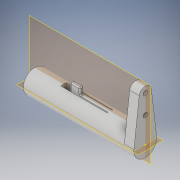
# Autodesk Inventor part: SR-T-07
Saved by Autodesk Inventor 2019.4 (Build 234330000, 330)
## iProperties
Created: 2019-06-15
Part Number: SR-T-07
Material: 一般
Document SubType Name: Modeling
Designer: Koki Shinjo
Mass: 0.853878 g
Surface Area: 9.79658 cm^2
Volume: 0.853878 cm^3
Density: 1 g/cm^3
Appearance: 既定
Author: Koki Shinjo
Autodesk Inventor part; units mm, degrees
ref_plane "YZ Plane" through (0, 0, 0) normal (1, 0, 0) x (0, 1, 0)
ref_plane "XY Plane" through (0, 0, 0) normal (0, 0, 1) x (1, 0, 0)
sketch "スケッチ1" plane through (0, 0, 0) normal (0, 0, 1) x (1, 0, 0)
  line L0 (0, 0) -> (0, 3)
  line L1 (0, 3) -> (-29, 3)
  line L2 (-29, 3) -> (-29, 0)
  line L3 (-29, 0) -> (0, 0)
  dimension "d0" = 29
  dimension "d1" = 3
  constraints: 8 end point, 3 perpendicular, 1 vertical
  measures "d0" distance of L0.end L1.end
  measures "d1" distance of L0.start L0.end
revolve "回転1" add sketch "スケッチ1" angle 360 about axis through (-29, 0, 0) along (1, 0, 0)
sketch "スケッチ2" plane through (0, 0, 0) normal (1, 0, 0) x (0, 0, -1)
  circle A0 centre (0, 6.7) radius 0.6
  circle A1 centre (0, 11.7) radius 0.6
  circle A2 centre (0, 11.7) radius 1.6
  line L0 (-1.5885, 11.8915) -> (-2.9784, 0.359)
  circle A3 centre (0, 0) radius 3 projected
  line L1 (2.9784, 0.359) -> (1.5885, 11.8915)
  dimension "d3" = 1.2
  dimension "d4" = 5
  dimension "d5" = 6.7
  dimension "d6" = 3.2
  constraints: 4 end point, 4 point on circle, 4 tangent, 3 centre point, 2 vertical alignment, 1 coincident, 1 equal radius
  measures "d3" diameter of A1
  measures "d4" distance of A1.centre A0.centre
  measures "d5" distance of point (0, 0) A0.centre
  measures "d6" diameter of A2
extrude "押し出し1" add sketch "スケッチ2" against normal blind 2.5 contours A2 | A2 L1 A3 L0
ref_plane "作業平面1" through (0, 0, 0) normal (0, 1, 0) x (-1, 0, 0)
sketch "スケッチ3" plane through (0, 0, 0) normal (0, 1, 0) x (-1, 0, 0)
  line L0 (0, 1.5885) -> (0, 2.9784) construction
  line L1 (0, 1.5885) -> (2.5, 1.5885) construction
  line L2 (2.5, 2.9784) -> (2.5, 1.5885) construction
  line L3 (2.5, 2.9784) -> (0, 2.9784) construction
  line L4 (0, 0.6) -> (2.5, 0.6) construction
  line L5 (0, 1.5885) -> (0, -1.5885) construction
  line L6 (0, -2.9784) -> (0, -1.5885) construction
  point P0 (0, 0)
sketch "スケッチ4" plane through (0, 0, 0) normal (0, 0, 1) x (1, 0, 0)
  line L0 (-29, 3) -> (-2.5, 3) projected
  line L1 (-19.2495, 3) -> (-16.6495, 3)
  line L2 (-16.6495, 3) -> (-16.6495, 4.8)
  line L3 (-16.6495, 4.8) -> (-19.2495, 4.8)
  line L4 (-19.2495, 4.8) -> (-19.2495, 3)
  line L5 (-19.4495, 3.871) -> (-14.8405, 3.871) construction
  line L6 (-19.4495, 4.8) -> (-19.4495, 3.871) construction
  line L7 (-19.4495, 4.8) -> (-16.4495, 4.8) construction
  line L8 (-16.4495, 4.8) -> (-14.8405, 3.871) construction
  line L9 (-16.6495, 3) -> (-19.2495, 3)
  line L10 (-19.2495, 3) -> (-19.2495, 2)
  line L11 (-19.2495, 2) -> (-16.6495, 2)
  line L12 (-16.6495, 2) -> (-16.6495, 3)
  point P0 (0, 0)
  dimension "d10" = 0.2
  dimension "d11" = 0
  dimension "d12" = 0.2
  dimension "d13" = 1
  constraints: 16 end point, 4 parallel, 2 horizontal, 2 perpendicular, 1 point on line
  measures "d10" distance between parallel lines of L6 L4
  measures "d11" distance between parallel lines of L7 L3
  measures "d12" distance from line of L7.end L2
  measures "d13" distance of L1.start L10.end
extrude "押し出し2" add sketch "スケッチ4" along normal mid plane 1
fillet "フィレット1" radius 0.5 2 edges at (-19.2495, 4.8, 0) (-16.6495, 4.8, 0)
fillet "フィレット2" radius 0.5 2 edges at (-16.6495, 2.9895, -0.2509) (-16.6495, 2.9895, 0.2509)
sketch "スケッチ5" plane through (-18.7495, 4.8, -0.5) normal (0, 1, 0) x (1, 0, 0)
  line L0 (0, -1) -> (-0.5, -1) projected
  line L1 (-0.5, -1) -> (9.5, -1)
  line L2 (9.5, -1) -> (9.5, 0) construction
  line L3 (9.5, 0) -> (-0.5, 0)
  line L4 (-0.5, 0) -> (-0.5, -1)
  line L5 (-0.5, 0) -> (0, 0) projected
  line L6 (9.7, -1.2) -> (-0.7, -1.2)
  line L7 (-0.7, -1.2) -> (-0.7, 0.2)
  line L8 (-0.7, 0.2) -> (9.7, 0.2)
  line L9 (9.7, 0.2) -> (9.7, -1.2) construction
  line L10 (9.5, -1) -> (9.5, -1.2)
  line L11 (9.5, 0) -> (9.5, 0.2)
  point P0 (18.7495, -0.5)
  dimension "d18" = 10
  dimension "d19" = 0.2
  constraints: 20 end point, 4 parallel, 4 point on line, 3 perpendicular, 1 horizontal, 3 other
  measures "d18" distance of L2.end L3.end
  measures "d19" distance between parallel lines of L1 L6
extrude "押し出し3" cut sketch "スケッチ5" against normal up to next
ref_plane "作業平面2" through (0, 0, 0) normal (0, 0, 1) x (1, 0, 0)
sketch "スケッチ6" plane through (0, 0, 0) normal (0, 0, 1) x (1, 0, 0)
  line L0 (-9.2495, 2.958) -> (-16.1495, 2.958) construction
  line L1 (-16.1495, 2.958) -> (-16.1495, 2.958) construction
  line L2 (-16.1495, 2.958) -> (-9.2495, 2.958) construction
  line L3 (-9.2495, 2.958) -> (-9.2495, 2.9172) construction
  line L4 (-9.2495, 2.9172) -> (-19.4495, 2.9172) construction
  line L5 (-19.4495, 2.9172) -> (-19.4495, 2.9172) construction
  line L6 (-19.4495, 2.9172) -> (-9.2495, 2.9172) construction
  line L7 (-9.2495, 2.9172) -> (-9.2495, 2.958) construction
  line L8 (-19.2495, -2.958) -> (-19.2495, -2.958) construction
  line L9 (-19.2495, -2.958) -> (-9.2495, -2.958) construction
  line L10 (-9.2495, -2.958) -> (-9.2495, -2.9172) construction
  line L11 (-9.2495, -2.9172) -> (-19.4495, -2.9172) construction
  line L12 (-19.4495, -2.9172) -> (-19.4495, -2.9172) construction
  line L13 (-19.4495, -2.9172) -> (-9.2495, -2.9172) construction
  line L14 (-9.2495, -2.9172) -> (-9.2495, -2.958) construction
  line L15 (-9.2495, -2.958) -> (-19.2495, -2.958) construction
  line L16 (-2.5, 0.359) -> (0, 0.359) construction
  line L17 (-2.5, 0.359) -> (-2.5, 0.359) construction
  line L18 (-2.5, 0.359) -> (0, 0.359) construction
  line L19 (0, 0.359) -> (0, 0.359) construction
  line L20 (-29, -3) -> (-29, 3) construction
  line L21 (-9.2495, -2.958) -> (-19.2495, -2.958) construction
  line L22 (-9.2495, 2.958) -> (-9.2495, -2.958) construction
  line L23 (-16.1495, 2.958) -> (-9.2495, 2.958) construction
  line L24 (-16.6495, 3.4641) -> (-16.6495, 4.3) construction
  arc A0 (-16.6495, 4.3) -> (-17.1495, 4.8) centre (-17.1495, 4.3) ccw construction
  line L25 (-17.1495, 4.8) -> (-18.7495, 4.8) construction
  arc A1 (-18.7495, 4.8) -> (-19.2495, 4.3) centre (-18.7495, 4.3) ccw construction
  line L26 (-19.2495, 4.3) -> (-19.2495, -2.958) construction
  line L27 (-19.2495, -3) -> (-19.2495, -2.958) projected
  line L28 (-19.2495, -3) -> (-9.2495, -3)
  line L29 (-9.2495, -3) -> (-9.2495, -1.5)
  line L30 (-9.2495, -1.5) -> (-19.2495, -1.5)
  line L31 (-19.2495, -1.5) -> (-19.2495, -3)
  line L32 (-9.2495, 2) -> (-16.6495, 2)
  line L33 (-16.6495, 2) -> (-16.6495, -0.5)
  line L34 (-16.6495, -0.5) -> (-9.2495, -0.5)
  line L35 (-9.2495, -0.5) -> (-9.2495, 2)
  line L36 (-29, 3) -> (-2.5, 3) construction
  point P0 (0, 0)
  dimension "d22" = 1.5
  dimension "d23" = 1
  dimension "d24" = 1
  constraints: 16 end point, 4 parallel, 3 point on line, 2 horizontal, 2 perpendicular, 1 other
  measures "d22" distance between parallel lines of L28 L30
  measures "d23" distance between parallel lines of L32 L36
  measures "d24" distance between parallel lines of L30 L34
extrude "押し出し4" cut sketch "スケッチ6" along normal mid plane 1
fillet "フィレット3" radius 0.5 6 edges at (-9.2495, -0.5, 0) (-9.2495, 2, 0) (-9.2495, -1.5, 0) (-16.6495, -0.5, 0) (-16.6495, 2, 0) (-19.2495, -1.5, 0)
move faces "移動1" translate (-2, 0, 0) faces at (-19.4495, -0.9724, -0.0765)
delete faces "削除1" heal yes whole lump no faces at (-17.1121, 4.7986, 0.1667) (-18.7869, 4.7986, 0.1667)
fillet "フィレット4" radius 0.3 2 edges at (-17.9495, 4.8, 0.5) (-17.9495, 4.8, -0.5)
delete faces "削除2" heal yes whole lump no faces at (-16.648, 3.4432, 0.3487)
delete faces "削除3" heal yes whole lump no faces at (-19.1825, -1.25, 0.1667)
delete faces "削除4" heal yes whole lump no faces at (-9.4995, -1.567, 0.1667)
fillet "フィレット5" radius 0.3 10 edges at (-16.6495, 4.7121, -0.4121) (-16.6495, 3.729, -0.5) (-16.6495, 4.7121, 0.4121) (-16.6495, 3.729, 0.5) (-16.6495, 4.8, 0) (-19.2495, 1.5, 0.5) (-19.2495, 4.8, 0) (-19.2495, 4.7121, -0.4121) (-19.2495, 1.5, -0.5) (-19.2495, 4.7121, 0.4121)
fillet "フィレット6" radius 0.3 4 edges at (-16.7392, 2.9713, 0.4139) (-16.7392, 2.9713, -0.4139) (-16.6495, 2.9983, -0.1001) (-16.6495, 2.9983, 0.1001)
fillet "フィレット7" radius 0.3 1 edges at (-9.2495, -1.5, 0)
